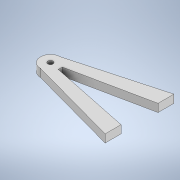
# Autodesk Inventor part: stojak
Saved by Autodesk Inventor 2020 (Build 240168000, 168)
## iProperties
Created: 2019-11-17
Part Number: stojak
Material: Ogólny
Document SubType Name: Modeling
Designer: Hubert Słomion
Density: 1 g/cm^3
Appearance: Domyślna
Author: Hubert Słomion
Autodesk Inventor part; units mm, degrees
ref_plane "YZ Plane" through (0, 0, 0) normal (1, 0, 0) x (0, 1, 0)
ref_plane "XZ Plane" through (0, 0, 0) normal (0, 1, 0) x (-1, 0, 0)
ref_plane "XY Plane" through (0, 0, 0) normal (0, 0, 1) x (1, 0, 0)
sketch "Szkic5" plane through (0, 0, 0) normal (0, 1, 0) x (-1, 0, 0)
  circle A0 centre (0, 0) radius 3.25
  circle A1 centre (0, 0) radius 5.5
  line L0 (0, 0) -> (0, 33.8176) construction
  line L1 (0, 0) -> (-112, 0) construction
  line L2 (0, 0) -> (112, 0) construction
  line L3 (0, 12.5) -> (-112, 43.2571)
  line L4 (-112, 43.2571) -> (-112, 23.2571)
  line L5 (0, -12.5) -> (-112, -43.2571)
  line L6 (-112, -43.2571) -> (-112, -23.2571)
  line L7 (-112, 23.2571) -> (-12.2389, 2.5414)
  line L8 (-112, -23.2571) -> (-12.2389, -2.5414)
  arc A2 (-12.2389, 2.5414) -> (-12.2389, -2.5414) centre (0, 0) ccw
  arc A3 (0, -12.5) -> (0, 12.5) centre (0, 0) ccw
  dimension "d7" = 6.5
  dimension "d8" = 11
  dimension "d12" = 112
  dimension "d13" = 180
  dimension "d14" = 20
  constraints: 18 end point, 4 centre point, 4 point on circle, 3 coincident, 3 symmetric about line, 2 horizontal, 2 vertical, 1 collinear, 1 point on line
  measures "d7" diameter of A0
  measures "d8" diameter of A1
  measures "d12" distance of L0.start L1.end
  measures "d13" angle of L1 L2
  measures "d14" distance of L3.end L4.end
extrude "Wyciągnięcie proste1" add sketch "Szkic5" along normal blind 10 contours A3 L5 L6 L8 A2 L7 L4 L3
sketch "Szkic6" plane through (0, 10, 0) normal (0, 1, 0) x (1, 0, 0)
  circle A0 centre (0, 0) radius 5.5
  circle A1 centre (0, 0) radius 3.25
  dimension "d17" = 6.5
  constraints: 2 centre point, 2 coincident
  measures "d17" diameter of A1
extrude "Wyciągnięcie proste2" add sketch "Szkic6" against normal blind 4
